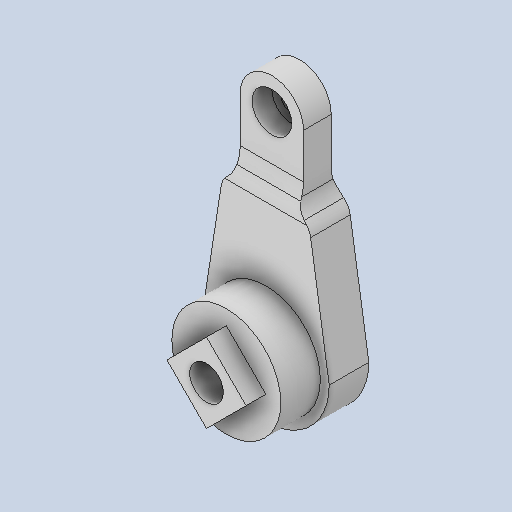
# Autodesk Inventor part: bièlle côté
Saved by Autodesk Inventor 2026.2 (Build 302298010, 298A)
## iProperties
Created: 2026-03-16
Part Number: bièlle côté
Material: Générique
Document SubType Name: Modeling
Designer: genon
Density: 1 g/cm^3
Appearance: Par défaut
Author: genon
Autodesk Inventor part; units mm, degrees
ref_plane "YZ Plane" through (0, 0, 0) normal (1, 0, 0) x (0, 1, 0)
ref_plane "XZ Plane" through (0, 0, 0) normal (0, 1, 0) x (-1, 0, 0)
sketch "Esquisse1" plane through (0, 0, 0) normal (1, 0, 0) x (0, 1, 0)
  circle A0 centre (0, 0) radius 16
  line L0 (-16, 0) -> (59, 0)
  line L1 (59, 0) -> (51, 0)
  circle A1 centre (51, 0) radius 5
  circle A2 centre (51, 0) radius 8
  line L2 (0, 16) -> (51, 8)
  line L3 (51, -8) -> (0, -16)
  circle A3 centre (0, 0) radius 11
  line L4 (34.396, -10.6045) -> (34.396, 10.6045)
  dimension "d0" = 32
  dimension "d1" = 75
  dimension "d2" = 8
  dimension "d3" = 10
  dimension "d4" = 16
  dimension "d5" = 22
  constraints: 10 end point, 5 point on circle, 4 centre point, 4 coincident, 3 point on line, 1 horizontal, 1 perpendicular
  measures "d0" diameter of A0
  measures "d1" distance of L0.start L0.end
  measures "d2" distance of L0.end L1.end
  measures "d3" diameter of A1
  measures "d4" diameter of A2
  measures "d5" diameter of A3
extrude "Extrusion1" add sketch "Esquisse1" along normal blind 10 contours L2 A0 L0 A3 | L0 A3 A0 L3 | L2 L4 L0 A0 | L0 L4 L3 A0
sketch "Esquisse2" plane through (0, 0, 0) normal (-1, 0, 0) x (0, 0, 1)
  circle A0 centre (0, 0) radius 11
  circle A1 centre (0, 0) radius 4.25
  dimension "d8" = 8.5
  constraints: 2 centre point, 2 coincident
  measures "d8" diameter of A1
extrude "Extrusion2" add sketch "Esquisse2" along normal blind 10
sketch "Esquisse3" plane through (-10, 0, 0) normal (-1, 0, 0) x (0, 0, 1)
  line L0 (0, 0) -> (-10, 0)
  circle A0 centre (0, 0) radius 11 projected
  line L1 (0, 0) -> (0, 10)
  circle A1 centre (0, 0) radius 4.25 projected
  line L2 (0, 0) -> (10, 0)
  line L3 (0, 0) -> (0, -10)
  line L4 (0, 10) -> (-10, 0)
  line L5 (0, 10) -> (10, 0)
  line L6 (10, 0) -> (0, -10)
  line L7 (-10, 0) -> (0, -10)
  circle A2 centre (0, 0) radius 4.25
  dimension "d12" = 10
  dimension "d13" = 10
  dimension "d14" = 10
  dimension "d15" = 10
  dimension "d16" = 8.5
  constraints: 16 end point, 2 horizontal, 2 vertical, 1 centre point, 1 coincident
  measures "d12" distance of L0.start L0.end
  measures "d13" distance of L1.start L1.end
  measures "d14" distance of L2.start L2.end
  measures "d15" distance of L2.start L3.end
  measures "d16" diameter of A2
extrude "Extrusion3" add sketch "Esquisse3" along normal blind 5 contours A1 L3 L7 L0 | L0 L4 L1 A1 | L1 L5 L2 A1 | L2 L6 L3 A1
sketch "Esquisse4" plane through (0, 0, 0) normal (-1, 0, 0) x (0, 0, 1)
  circle A0 centre (0, 0) radius 13.75
  circle A1 centre (0, 0) radius 11
  dimension "d19" = 27.5
  constraints: 2 centre point, 2 coincident
  measures "d19" diameter of A0
extrude "Extrusion4" add sketch "Esquisse4" along normal up to surface (10 mm away)
ref_plane "Plan de construction1" through (5, 0, 0) normal (-1, 0, 0) x (0, 0, 1)
sketch "Esquisse7" plane through (5, 0, 0) normal (-1, 0, 0) x (0, 0, 1)
  point P0 (0, 0)
sketch "Esquisse8" plane through (5, 0, 0) normal (-1, 0, 0) x (0, 0, 1)
  circle A0 centre (0, 51) radius 5 projected
  circle A1 centre (0, 51) radius 4.25 projected
  line L0 (-16, 0) -> (-10.6045, 34.396) projected
  line L1 (10.6045, 34.396) -> (16, 0) projected
  arc A2 (8, 51) -> (-8, 51) centre (0, 51) ccw projected
  line L2 (-10.6045, 34.396) -> (10.6045, 34.396) projected
  line L3 (-10.6045, 34.396) -> (-8, 51)
  line L4 (8, 51) -> (10.6045, 34.396)
  line L5 (10.6045, 34.396) -> (-10.6045, 34.396)
  point P0 (0, 0)
  constraints: 6 end point, 1 horizontal
extrude "Extrusion6" add sketch "Esquisse8" along normal mid plane 7 contours L4 L2 L3 A2
sketch "Esquisse9" plane through (8.5, 0, 0) normal (1, 0, 0) x (0, 0, -1)
  circle A0 centre (0, 51) radius 5 projected
  circle A1 centre (0, 51) radius 2.75
  circle A2 centre (0, 51) radius 5
  point P0 (0, 0)
  dimension "d37" = 5.5
  constraints: 2 centre point, 2 coincident, 1 concentric
  measures "d37" diameter of A1
extrude "Extrusion7" add sketch "Esquisse9" against normal blind 2
fillet "Congé1" radius 10 4 edges at (8.5, 34.396, 0) (1.5, 34.396, 0) (10, 34.396, 0) (0, 34.396, 0)
sketch "Esquisse10" plane through (0, 0, 0) normal (-1, 0, 0) x (0, 0, 1)
  line L0 (-10.9703, 32.0645) -> (10.9703, 32.0645) projected
  line L1 (-10.9703, 32.0645) -> (10.9703, 32.0645)
  arc A0 (8, 51) -> (-8, 51) centre (0, 51) ccw projected
  line L2 (-8, 51) -> (-8, 32.0645)
  line L3 (9.7782, 39.6638) -> (8, 51) projected
  line L4 (8, 51) -> (8, 32.0645)
  arc A1 (8, 51) -> (-8, 51) centre (0, 51) ccw
  line L5 (-10.9703, 32.0645) -> (-8, 51)
  line L6 (8, 51) -> (10.9703, 32.0645)
  point P0 (0, 0)
  constraints: 10 end point, 2 collinear, 2 point on circle, 2 point on line, 2 tangent, 1 centre point, 1 perpendicular, 1 vertical
extrude "Extrusion8" cut sketch "Esquisse10" against normal blind 10 contours L5 L2 L0 | L4 L3 L6 L0
fillet "Congé2" radius 5 2 edges at (5, 32.0645, -8) (5, 32.0645, -10.9703)
fillet "Congé3" radius 5 2 edges at (5, 32.0645, 10.9703) (5, 32.0645, 8)
